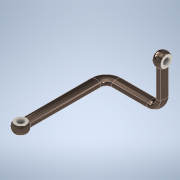
# Autodesk Inventor part: Part15 3D Sketches
Saved by Autodesk Inventor 2022.2 (Build 262287010, 287A)
## iProperties
Created: 2022-12-16
Part Number: Part15 3D Sketches
Material: Steel, Carbon
Document SubType Name: Modeling
Designer: User
Mass: 1921.04 g
Surface Area: 462.473 cm^2
Volume: 244.719 cm^3
Density: 7.85 g/cm^3
Appearance: Gunmetal - Antique Polished
Author: User
Autodesk Inventor part; units mm, degrees
ref_plane "YZ Plane" through (0, 0, 0) normal (1, 0, 0) x (0, 1, 0)
ref_plane "XZ Plane" through (0, 0, 0) normal (0, 1, 0) x (-1, 0, 0)
ref_plane "XY Plane" through (0, 0, 0) normal (0, 0, 1) x (1, 0, 0)
sketch "Sketch1" plane through (0, 0, 0) normal (0, 0, -1) x (-1, 0, 0)
  line L0 (8, 0) -> (-8, 0) construction
  arc A0 (11.7333, -5.9213) -> (11.7333, 5.9213) centre (8, 0) ccw
  arc A1 (-11.7333, 5.9213) -> (-11.7333, -5.9213) centre (-8, 0) ccw
  arc A2 (11.7333, 5.9213) -> (-11.7333, 5.9213) centre (0, -12.6886) ccw
  arc A3 (-11.7333, -5.9213) -> (11.7333, -5.9213) centre (0, 12.6886) ccw
  point P0 (0, 0)
  point P1 (0, 0)
  dimension "d7" = 16
  dimension "d8" = 7
  dimension "d9" = 22
  constraints: 8 point on circle, 4 centre point, 3 coincident, 3 symmetric about line, 2 end point, 2 tangent, 1 equal radius, 1 horizontal, 1 midpoint, 1 vertical alignment, 1 other
  measures "d7" distance of L0.start L0.end
  measures "d8" radius of A0
  measures "d9" radius of A2
sketch3d "3D Sketch1"
  line L0 (0, 0, 0) -> (0, 0, -214)
  arc A0 (0, 0, -214) -> (30, 0, -244) centre (30, 0, -214) ccw
  line L1 (30, 0, -244) -> (130, 0, -244)
  arc A1 (130, 0, -244) -> (160, 30, -244) centre (130, 30, -244) ccw
  line L2 (160, 30, -244) -> (160, 123, -244)
  dimension "d0" = 244
  dimension "d3" = 123
  dimension "d4" = 160
  dimension "d5" = 30
  dimension "d6" = 30
sweep "Sweep1" add profiles "Sketch1" path "3D Sketch1"
sketch "Sketch2" plane through (0, 0, 0) normal (0, 0, -1) x (-1, 0, 0)
  arc A0 (16.3631, -11.5) -> (16.3631, 11.5) centre (0, 0) ccw
  line L0 (0, 20) -> (0, -20) construction
  line L1 (16.3631, 11.5) -> (0, 11.5)
  line L2 (16.3631, -11.5) -> (0, -11.5)
  line L3 (0, 11.5) -> (0, -11.5)
  dimension "d12" = 20
  dimension "d13" = 23
  constraints: 8 end point, 2 parallel, 2 point on circle, 2 point on line, 2 vertical, 1 centre point, 1 coincident, 1 midpoint, 1 perpendicular
  measures "d12" radius of A0
  measures "d13" distance between parallel lines of L2 L1
revolve "Revolution1" add sketch "Sketch2" angle 360 about axis through (0, 20, 0) along (0, -1, 0)
sketch "Sketch3" plane through (160, 123, -236) normal (0, 1, 0) x (1, 0, 0)
  arc A0 (5.9213, 19.7333) -> (-5.9213, 19.7333) centre (0, 16) ccw projected
  arc A1 (11.5, 24.0936) -> (-11.5, 24.0936) centre (0, 7.7305) ccw
  line L0 (-11.5, 7.7305) -> (11.5, 7.7305)
  line L1 (-11.5, 7.7305) -> (-11.5, 24.0936)
  line L2 (11.5, 24.0936) -> (11.5, 7.7305)
  point P0 (-160, -236)
  point P1 (0, 7.7305)
  dimension "d15" = 20
  dimension "d16" = 23
  constraints: 6 end point, 2 midpoint, 2 point on circle, 1 centre point, 1 horizontal, 1 parallel, 1 perpendicular, 1 vertical, 1 vertical alignment
  measures "d15" radius of A1
  measures "d16" distance between parallel lines of L2 L1
revolve "Revolution2" add sketch "Sketch3" angle 360 about axis through (148.5, 123, -243.7305) along (1, 0, 0)
sketch "Sketch4" plane through (0, 11.5, 0) normal (0, 1, 0) x (1, 0, 0)
  circle A0 centre (0, 0) radius 16.3631 projected
  point P0 (0, 0)
  constraints: 1 coincident
hole "Hole1" at (0, 11.5, 0) direction (0, -1, 0) diameter 18 end through all
sketch "Sketch5" plane through (171.5, 123, -243.7305) normal (1, 0, 0) x (0, 0, -1)
  circle A0 centre (0, 0) radius 16.3631 projected
  point P0 (-243.7305, -123)
  constraints: 1 coincident
hole "Hole2" at (171.5, 123, -243.7305) direction (-1, 0, 0) diameter 18 end through all
ref_plane "Work Plane1" through (0, 0, 0) normal (0, 0, -1) x (-1, 0, 0)
equation "\"d6\" = d5"
body "Solid1"
